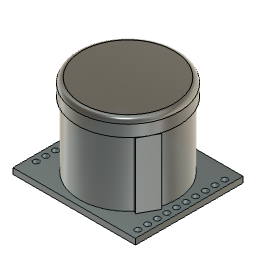
ZE15-CO v1 (Autodesk Fusion 360 design; units mm, degrees)
Autodesk Fusion 360 part; units mm, degrees
sketch "Sketch1" plane through (0, 0, 0) normal (0, 0, 1) x (1, 0, 0)
  line L0 (-12.7, 11.15) -> (12.7, 11.15)
  line L1 (12.7, 11.15) -> (12.7, -11.15)
  line L2 (12.7, -11.15) -> (-12.7, -11.15)
  line L3 (-12.7, -11.15) -> (-12.7, 11.15)
  line L4 (0, 0) -> (0, 28.3109) construction
  line L5 (0, 0) -> (22.2982, 0) construction
  circle A0 centre (11.4, 8.65) radius 0.6
  circle A1 centre (11.4, 6.65) radius 0.6
  circle A2 centre (11.4, 4.65) radius 0.6
  circle A3 centre (11.4, 2.65) radius 0.6
  circle A4 centre (11.4, 0.65) radius 0.6
  circle A5 centre (11.4, -1.35) radius 0.6
  circle A6 centre (11.4, -3.35) radius 0.6
  circle A7 centre (11.4, -5.35) radius 0.6
  circle A8 centre (11.4, -7.35) radius 0.6
  circle A9 centre (11.4, -9.35) radius 0.6
  circle A10 centre (-11.4, 0.35) radius 0.6
  circle A11 centre (-11.4, -1.65) radius 0.6
  circle A12 centre (-11.4, -3.65) radius 0.6
  circle A13 centre (-11.4, -5.65) radius 0.6
  circle A14 centre (-11.4, -7.65) radius 0.6
  circle A15 centre (-11.4, 9.85) radius 0.6
  circle A16 centre (-11.4, 7.85) radius 0.6
  circle A17 centre (-11.4, 5.85) radius 0.6
  circle A18 centre (-11.4, 3.85) radius 0.6
  dimension "d1" = 22.3
  dimension "d2" = 25.4
  dimension "d3" = 2.5
  dimension "d4" = 1.2
  dimension "d5" = 1.3
  dimension "d8" = 0
  dimension "d9" = -18
  dimension "d10" = 1.2
  dimension "d11" = 1.3
  dimension "d12" = 10.8
  dimension "d15" = 0
  dimension "d16" = -8
  dimension "d17" = 1.2
  dimension "d18" = 1.3
  dimension "d19" = 1.3
  dimension "d22" = 0
  dimension "d23" = -6
  constraint horizontal L0
  constraint vertical L1
  constraint horizontal L2
  constraint vertical L3
  constraint coincident L4.start L5.start
  constraint perpendicular L0 L4
  constraint symmetric L1 L3 L4
  constraint perpendicular L4 L5
  constraint symmetric L0 L2 L5
  measures "d1" distance of L0.start L2.end
  measures "d2" distance of L1 L3
  measures "d3" distance of L0 A0.centre
  measures "d4" diameter of A0
  measures "d5" distance of L1 A0.centre
  measures "d10" diameter of A10
  measures "d11" distance of L3 A10.centre
  measures "d12" distance of L0 A10.centre
  measures "d17" diameter of A15
  measures "d18" distance of L0 A15.centre
  measures "d19" distance of L3 A15.centre
extrude "Extrude1" add sketch "Sketch1" along normal blind 1.2
sketch "Sketch2" plane through (0, 0, 1.2) normal (0, 0, 1) x (-1, 0, 0)
  circle A0 centre (11.4, 5.65) radius 0.6
  circle A1 centre (-11.4, -8.65) radius 0.6
  circle A2 centre (11.4, -9.85) radius 0.6
  circle A3 centre (11.4, 3.65) radius 0.6
  circle A4 centre (-11.4, -4.65) radius 0.6
  circle A5 centre (-11.4, -6.65) radius 0.6
  circle A6 centre (11.4, 7.65) radius 0.6
  circle A7 centre (11.4, -0.35) radius 0.6
  circle A8 centre (-11.4, 5.35) radius 0.6
  circle A9 centre (-11.4, 7.35) radius 0.6
  circle A10 centre (-11.4, -0.65) radius 0.6
  circle A11 centre (-11.4, 9.35) radius 0.6
  circle A12 centre (-11.4, -2.65) radius 0.6
  circle A13 centre (-11.4, 3.35) radius 0.6
  circle A14 centre (11.4, -7.85) radius 0.6
  circle A15 centre (11.4, -5.85) radius 0.6
  circle A16 centre (11.4, -3.85) radius 0.6
  circle A17 centre (11.4, 1.65) radius 0.6
  circle A18 centre (-11.4, 1.35) radius 0.6
  line L0 (12.7, 11.15) -> (-12.7, 11.15)
  line L1 (-12.7, 11.15) -> (-12.7, -11.15)
  line L2 (-12.7, -11.15) -> (12.7, -11.15)
  line L3 (12.7, -11.15) -> (12.7, 11.15)
  circle A19 centre (0, 0) radius 10
  dimension "d26" = 20
  constraint coincident A19.centre origin
  measures "d26" diameter of A19
extrude "Extrude2" add sketch "Sketch2" along normal blind 13.6 contours A19
ref_plane "WorkPlane1" through (0, 0, 14.8) normal (0, 0, 1) x (-1, 0, 0)
sketch "Sketch3" plane through (0, 0, 14.8) normal (0, 0, 1) x (1, 0, 0)
  circle A0 centre (0, 0) radius 10.5
  dimension "d30" = 21
  constraint coincident A0.centre origin
  measures "d30" diameter of A0
extrude "Extrude3" add sketch "Sketch3" along normal blind 3.4
fillet "Fillet1" radius 1 1 edges at (-9.7894, -3.797, 18.2)
sketch "Sketch4" plane through (0, 0, 1.2) normal (0, 0, 1) x (-1, 0, 0)
  circle A0 centre (0, 0) radius 10
  circle A1 centre (11.4, 5.65) radius 0.6
  circle A2 centre (-11.4, -8.65) radius 0.6
  circle A3 centre (11.4, -9.85) radius 0.6
  circle A4 centre (11.4, 3.65) radius 0.6
  circle A5 centre (-11.4, -4.65) radius 0.6
  circle A6 centre (-11.4, -6.65) radius 0.6
  circle A7 centre (11.4, 7.65) radius 0.6
  circle A8 centre (11.4, -0.35) radius 0.6
  circle A9 centre (-11.4, 5.35) radius 0.6
  circle A10 centre (-11.4, 7.35) radius 0.6
  circle A11 centre (-11.4, -0.65) radius 0.6
  circle A12 centre (-11.4, 9.35) radius 0.6
  circle A13 centre (-11.4, -2.65) radius 0.6
  circle A14 centre (-11.4, 3.35) radius 0.6
  circle A15 centre (11.4, -7.85) radius 0.6
  circle A16 centre (11.4, -5.85) radius 0.6
  circle A17 centre (11.4, -3.85) radius 0.6
  circle A18 centre (11.4, 1.65) radius 0.6
  circle A19 centre (-11.4, 1.35) radius 0.6
  line L0 (12.7, 11.15) -> (-12.7, 11.15)
  line L1 (-12.7, 11.15) -> (-12.7, -11.15)
  line L2 (-12.7, -11.15) -> (12.7, -11.15)
  line L3 (12.7, -11.15) -> (12.7, 11.15)
ref_plane "WorkPlane2" through (0, 0, 14.8) normal (0, 0, -1) x (-1, 0, 0)
sketch "Sketch5" plane through (0, 0, 14.8) normal (0, 0, -1) x (-1, 0, 0)
ref_plane "WorkPlane3" through (0, 0, 14.8) normal (0, 0, -1) x (-1, 0, 0)
sketch "Sketch6" plane through (0, 0, 14.8) normal (0, 0, -1) x (-1, 0, 0)
  line L0 (-9.3153, -2.737) -> (-7.4198, -6.2594)
  line L1 (-7.4198, -6.2594) -> (-8.3004, -6.7333)
  line L2 (-8.3004, -6.7333) -> (-10.1959, -3.2109)
  line L3 (-10.1959, -3.2109) -> (-9.3153, -2.737)
  circle A0 centre (0, 0) radius 9.5
  dimension "d37" = 4
  dimension "d38" = 1
  dimension "d39" = 4
  constraint perpendicular L0 L1
  constraint perpendicular L1 L2
  constraint tangent L0 A0
  measures "d37" distance of L0.start L0.end
  measures "d38" distance of L0.end L1.end
  measures "d39" distance of L1.end L2.end
extrude "Extrude4" add sketch "Sketch6" along normal blind 13.6 contours L0 L1 L2 L3
sketch "Sketch7" plane through (0, 0, 0) normal (0, 0, -1) x (1, 0, 0)
  circle A0 centre (-11.4, 5.65) radius 0.6
  circle A1 centre (11.4, -8.65) radius 0.6
  circle A2 centre (-11.4, -9.85) radius 0.6
  circle A3 centre (-11.4, 3.65) radius 0.6
  circle A4 centre (11.4, -4.65) radius 0.6
  circle A5 centre (11.4, -6.65) radius 0.6
  circle A6 centre (-11.4, 7.65) radius 0.6
  circle A7 centre (-11.4, -0.35) radius 0.6
  circle A8 centre (11.4, 5.35) radius 0.6
  circle A9 centre (11.4, 7.35) radius 0.6
  circle A10 centre (11.4, -0.65) radius 0.6
  circle A11 centre (11.4, 9.35) radius 0.6
  circle A12 centre (11.4, -2.65) radius 0.6
  circle A13 centre (11.4, 3.35) radius 0.6
  circle A14 centre (-11.4, -7.85) radius 0.6
  circle A15 centre (-11.4, -5.85) radius 0.6
  circle A16 centre (-11.4, -3.85) radius 0.6
  circle A17 centre (-11.4, 1.65) radius 0.6
  circle A18 centre (11.4, 1.35) radius 0.6
  line L0 (12.7, 11.15) -> (-12.7, 11.15)
  line L1 (-12.7, 11.15) -> (-12.7, -11.15)
  line L2 (-12.7, -11.15) -> (12.7, -11.15)
  line L3 (12.7, -11.15) -> (12.7, 11.15)
